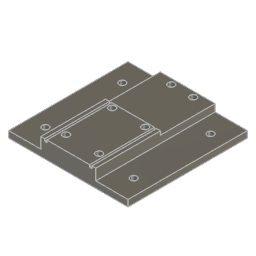
x_stage (Autodesk Fusion 360 design; units mm, degrees)
part number: 2026-04-23-15-36-49-562
Autodesk Fusion 360 part; units mm, degrees
note: some values were not read from the file. Chosen so that the rebuilt part matches the saved one: which face or edge a step refers to. Set by a fixed rule: which sketch regions a step uses.
sketch "Sketch1" plane through (0, 0, 0) normal (0, 0, 1) x (1, 0, 0)
  line L0 (-27.2, 27.2) -> (27.2, 27.2)
  line L1 (27.2, 27.2) -> (27.2, -27.2)
  line L2 (27.2, -27.2) -> (-27.2, -27.2)
  line L3 (-27.2, -27.2) -> (-27.2, 27.2)
  line L4 (-27.2, 27.2) -> (27.2, -27.2) construction
  line L5 (27.2, 27.2) -> (-27.2, -27.2) construction
  circle A0 centre (-20.1, 17.5) radius 1.5
  circle A1 centre (-20.1, -17.5) radius 1.5
  circle A2 centre (20.1, 17.5) radius 1.5
  circle A3 centre (20.1, -17.5) radius 1.5
  circle A4 centre (-4, 24.95) radius 1.5
  circle A5 centre (4, 24.95) radius 1.5
  circle A6 centre (-4, 7.95) radius 1.5
  circle A7 centre (4, 7.95) radius 1.5
  circle A8 centre (0, 10.7) radius 1.5
  dimension "d1" = 54.4
  dimension "d2" = 3
  dimension "d3" = 35
  dimension "d4" = 9.7
  dimension "d9" = 3
  dimension "d10" = 24.95
  dimension "d11" = 4
  dimension "d12" = 4
  dimension "d19" = 7.1
  dimension "d20" = 7.1
  dimension "d21" = 17
  dimension "d22" = 16.5
  dimension "d23" = 3
  constraint horizontal L0
  constraint perpendicular L0 L1
  constraint parallel L0 L2
  constraint parallel L1 L3
  constraint coincident L4 origin
  constraint coincident L5 origin
  constraint equal L0 L3
  constraint vertical A0.centre A1.centre
  constraint horizontal A1.centre A3.centre
  constraint vertical A2.centre A3.centre
  constraint horizontal A0.centre A2.centre
  constraint equal A0 A1
  constraint equal A1 A3
  constraint equal A2 A3
  constraint equal A4 A5
  constraint horizontal A4.centre A5.centre
  constraint vertical A5.centre A7.centre
  constraint vertical A4.centre A6.centre
  constraint equal A4 A6
  constraint equal A6 A7
  constraint horizontal A6.centre A7.centre
  constraint vertical origin A8.centre
  measures "d1" distance of L0.start L0.end
  measures "d2" diameter of A0
  measures "d3" distance of A0.centre A1.centre
  measures "d4" distance of L0 A0.centre
  measures "d9" diameter of A4
  measures "d10" vertical distance of origin A4.centre
  measures "d11" horizontal distance of origin A4.centre
  measures "d12" horizontal distance of origin A5.centre
  measures "d19" distance of L3 A0.centre
  measures "d20" distance of L1 A2.centre
  measures "d21" distance of A4.centre A6.centre
  measures "d22" distance of L0 A8.centre
  measures "d23" diameter of A8
extrude "Extrude1" add sketch "Sketch1" along normal blind 3 contours L0 L1 L2 L3 | A4 | A5 | A6 | A7 | A8
sketch "Sketch2" plane through (0, 0, 3) normal (0, 0, 1) x (-1, 0, 0)
  circle A0 centre (-20.1, 17.5) radius 1.5
  circle A1 centre (20.1, -17.5) radius 1.5
  circle A2 centre (20.1, 17.5) radius 1.5
  circle A3 centre (-20.1, -17.5) radius 1.5
  line L0 (27.2, 27.2) -> (-27.2, 27.2)
  line L1 (-27.2, 27.2) -> (-27.2, -27.2)
  line L2 (-27.2, -27.2) -> (27.2, -27.2)
  line L3 (27.2, -27.2) -> (27.2, 27.2)
  line L4 (12.5, -27.2) -> (-12.5, -27.2)
  line L5 (-12.5, -27.2) -> (-12.5, 27.2)
  line L6 (-12.5, 27.2) -> (12.5, 27.2)
  line L7 (12.5, 27.2) -> (12.5, -27.2)
  line L8 (12.5, -27.2) -> (-12.5, 27.2) construction
  line L9 (-12.5, -27.2) -> (12.5, 27.2) construction
  dimension "d13" = 25
  constraint horizontal L4
  constraint perpendicular L4 L5
  constraint parallel L4 L6
  constraint parallel L5 L7
  constraint coincident L8 origin
  constraint coincident L9 origin
  constraint coincident L2 L4.start
  measures "d13" distance of L4.start L4.end
extrude "Extrude2" add sketch "Sketch2" along normal blind 3 contours L0 L2 L4 L5 L6 L7
sketch "Sketch5" plane through (0, 0, 6) normal (0, 0, 1) x (-1, 0, 0)
  line L0 (12.5, 27.2) -> (-12.5, 27.2)
  line L1 (-12.5, 27.2) -> (-12.5, -27.2)
  line L2 (-12.5, -27.2) -> (12.5, -27.2)
  line L3 (12.5, -27.2) -> (12.5, 27.2)
  circle A0 centre (7.5, -0.3) radius 1.5
  circle A1 centre (-7.5, -0.3) radius 1.5
  circle A2 centre (7.5, 20.7) radius 1.5
  circle A3 centre (-7.5, 20.7) radius 1.5
  circle A4 centre (5, -24.7) radius 1.5
  circle A5 centre (-5, -24.7) radius 1.5
  circle A6 centre (5, -10.7) radius 1.5
  circle A7 centre (-5, -10.7) radius 1.5
  dimension "d27" = 15
  dimension "d28" = 21
  dimension "d29" = 3
  dimension "d31" = 7.5
  dimension "d34" = 10
  dimension "d35" = 14
  dimension "d36" = 3
  dimension "d37" = 5
  dimension "d38" = 2.5
  dimension "d49" = 26.9
  constraint vertical A0.centre A2.centre
  constraint horizontal A0.centre A1.centre
  constraint horizontal A2.centre A3.centre
  constraint vertical A1.centre A3.centre
  constraint equal A2 A3
  constraint equal A0 A2
  constraint equal A0 A1
  constraint vertical A4.centre A6.centre
  constraint horizontal A6.centre A7.centre
  constraint vertical A5.centre A7.centre
  constraint horizontal A4.centre A5.centre
  constraint equal A4 A5
  constraint equal A5 A7
  constraint equal A6 A7
  measures "d27" distance of A0.centre A1.centre
  measures "d28" distance of A0.centre A2.centre
  measures "d29" diameter of A0
  measures "d31" horizontal distance of origin A2.centre
  measures "d34" distance of A4.centre A5.centre
  measures "d35" vertical distance of A4.centre A6.centre
  measures "d36" diameter of A4
  measures "d37" horizontal distance of origin A4.centre
  measures "d38" distance of L2 A4.centre
  measures "d49" distance of L2 A0.centre
extrude "Extrude5" cut sketch "Sketch5" against normal blind 3 contours A0 | A1 | A2 | A3 | A4 | A5
sketch "Sketch6" plane through (0, 0, 6) normal (0, 0, 1) x (-1, 0, 0)
  line L0 (12.5, 27.2) -> (-12.5, 27.2)
  line L1 (-12.5, 27.2) -> (-12.5, -27.2)
  line L2 (-12.5, -27.2) -> (12.5, -27.2)
  line L3 (12.5, -27.2) -> (12.5, 27.2)
  circle A0 centre (5, -24.7) radius 1.5
  circle A1 centre (7.5, 20.7) radius 1.5
  circle A2 centre (7.5, -0.3) radius 1.5
  circle A3 centre (-5, -24.7) radius 1.5
  circle A4 centre (-7.5, 20.7) radius 1.5
  circle A5 centre (-7.5, -0.3) radius 1.5
  line L4 (12.5, 27.2) -> (-12.5, 27.2)
  line L5 (-12.5, 27.2) -> (-12.5, -2.3)
  line L6 (-12.5, -2.3) -> (12.5, -2.3)
  line L7 (12.5, -2.3) -> (12.5, 27.2)
  dimension "d39" = 29.5
  constraint horizontal L4
  constraint vertical L5
  constraint horizontal L6
  constraint vertical L7
  constraint coincident L1 L5.end
  constraint coincident L0.start L3.end
  measures "d39" distance of L0.start L6.end
extrude "Extrude6" add sketch "Sketch6" along normal blind 2 contours L0 L1 L3 L4 L5 L6 L7
extrude "Extrude8" add 1 faces at (1.484, 9.3012, 6) along direction (0, 0, 1) blind 0.3
sketch "Sketch8" plane through (0, 0, 8) normal (0, 0, 1) x (-1, 0, 0)
  circle A0 centre (7.5, -0.3) radius 1.5
  circle A1 centre (7.5, 20.7) radius 1.5
  circle A2 centre (-7.5, 20.7) radius 1.5
  circle A3 centre (-7.5, -0.3) radius 1.5
  line L0 (12.5, -2.3) -> (12.5, 27.2)
  line L1 (12.5, 27.2) -> (-12.5, 27.2)
  line L2 (-12.5, 27.2) -> (-12.5, -2.3)
  line L3 (-12.5, -2.3) -> (12.5, -2.3)
  line L4 (10.73, -2.3) -> (9.73, -2.3)
  line L5 (9.73, -2.3) -> (9.73, 27.2)
  line L6 (9.73, 27.2) -> (10.73, 27.2)
  line L7 (10.73, 27.2) -> (10.73, -2.3)
  line L8 (-9.73, -2.3) -> (-10.73, -2.3)
  line L9 (-10.73, -2.3) -> (-10.73, 27.2)
  line L10 (-10.73, 27.2) -> (-9.73, 27.2)
  line L11 (-9.73, 27.2) -> (-9.73, -2.3)
  dimension "d52" = 1
  dimension "d53" = 1.77
  dimension "d54" = 1.77
  constraint horizontal L4
  constraint vertical L5
  constraint horizontal L6
  constraint vertical L7
  constraint coincident L1 L5.end
  constraint coincident L3 L4.start
  constraint horizontal L8
  constraint vertical L9
  constraint horizontal L10
  constraint vertical L11
  constraint coincident L1 L9.end
  constraint coincident L3 L8.start
  constraint equal L4 L8
  measures "d52" distance of L4.start L4.end
  measures "d53" distance of L0 L7
  measures "d54" distance of L2 L9
extrude "Extrude9" cut sketch "Sketch8" against normal blind 1 contours L1 L3 L4 L5 L6 L7 | L1 L3 L8 L9 L10 L11
sketch "Sketch9" plane through (0, 0, 0) normal (0, 0, -1) x (1, 0, 0)
  circle A0 centre (20.1, 17.5) radius 1.5
  circle A1 centre (-20.1, 17.5) radius 1.5
  circle A2 centre (20.1, -17.5) radius 1.5
  circle A3 centre (-20.1, -17.5) radius 1.5
  line L0 (27.2, 27.2) -> (-27.2, 27.2)
  line L1 (-27.2, 27.2) -> (-27.2, -27.2)
  line L2 (-27.2, -27.2) -> (27.2, -27.2)
  line L3 (27.2, -27.2) -> (27.2, 27.2)
  line L4 (20.2, 15.2) -> (34.2, 15.2)
  arc A4 (34.2, 15.2) -> (34.2, 27.2) centre (34.2, 21.2) ccw
  line L5 (34.2, 27.2) -> (20.2, 27.2)
  arc A5 (20.2, 27.2) -> (20.2, 15.2) centre (20.2, 21.2) ccw
  line L6 (20.2, 21.2) -> (34.2, 21.2) construction
  circle A6 centre (34.2, 21.2) radius 3.125
  line L7 (0, 0) -> (0, -11.2612) construction
  line L8 (0, 0) -> (-11.04, 0) construction
  line L9 (0, 0) -> (0, -11.2612) construction
  circle A7 centre (-34.2, 21.2) radius 3.125
  arc A8 (-20.2, 15.2) -> (-20.2, 27.2) centre (-20.2, 21.2) ccw
  arc A9 (-34.2, 27.2) -> (-34.2, 15.2) centre (-34.2, 21.2) ccw
  line L10 (-34.2, 27.2) -> (-20.2, 27.2)
  line L11 (-20.2, 21.2) -> (-34.2, 21.2) construction
  line L12 (-20.2, 15.2) -> (-34.2, 15.2)
  circle A10 centre (-20.1, 17.5) radius 1.5
  line L13 (20.2, -21.2) -> (34.2, -21.2) construction
  line L14 (34.2, -27.2) -> (20.2, -27.2)
  arc A11 (34.2, -27.2) -> (34.2, -15.2) centre (34.2, -21.2) ccw
  arc A12 (20.2, -15.2) -> (20.2, -27.2) centre (20.2, -21.2) ccw
  line L15 (20.2, -15.2) -> (34.2, -15.2)
  circle A13 centre (20.1, -17.5) radius 1.5
  circle A14 centre (34.2, -21.2) radius 3.125
  line L16 (-20.2, -15.2) -> (-34.2, -15.2)
  arc A15 (-20.2, -27.2) -> (-20.2, -15.2) centre (-20.2, -21.2) ccw
  arc A16 (-34.2, -15.2) -> (-34.2, -27.2) centre (-34.2, -21.2) ccw
  circle A17 centre (-34.2, -21.2) radius 3.125
  circle A18 centre (-20.1, -17.5) radius 1.5
  line L17 (-20.2, -21.2) -> (-34.2, -21.2) construction
  line L18 (-34.2, -27.2) -> (-20.2, -27.2)
  circle A19 centre (-20.1, -17.5) radius 1.5
  point P0 (27.2, 21.2)
  point P1 (-27.2, 27.2)
  point P2 (-27.2, 21.2)
  point P3 (27.2, -27.2)
  point P4 (27.2, -21.2)
  point P5 (-27.2, -21.2)
  point P6 (-27.2, -27.2)
  point P7 (-27.2, -27.2)
  dimension "d62" = 6
  dimension "d63" = 6.25
  dimension "d64" = 6
  dimension "d65" = 7
  constraint tangent L4 A4
  constraint tangent A4 L5
  constraint parallel L4 L5
  constraint tangent L5 A5
  constraint tangent L4 A5
  constraint perpendicular L3 L6
  constraint coincident L3 P0
  constraint midpoint L6 P0
  constraint concentric A4 A6
  constraint coincident L7.start L8.start
  constraint vertical L7
  constraint perpendicular L7 L8
  constraint symmetric A0 L7 A10
  constraint symmetric L0.start L7 P1
  constraint symmetric L4.start L7 A8.start
  constraint symmetric L4.end L7 A9.end
  constraint symmetric A4.end L7 A9.start
  constraint symmetric L5.end L7 A8.end
  constraint symmetric A4 L7 A9
  constraint symmetric A5 L7 A8
  constraint symmetric P0 L7 P2
  constraint symmetric A6 L7 A7
  constraint symmetric L8.start L7 L9.start
  constraint symmetric L9.end L7 L7.end
  constraint symmetric A0 L8 A13
  constraint symmetric A1 L8 A19
  constraint symmetric L0.start L8 P3
  constraint symmetric P1 L8 P7
  constraint symmetric L4.start L8 A12.start
  constraint symmetric L4.end L8 A11.end
  constraint symmetric A4.end L8 L14.start
  constraint symmetric L5.end L8 L14.end
  constraint symmetric A4 L8 A11
  constraint symmetric A5 L8 A12
  constraint symmetric P0 L8 P4
  constraint symmetric A6 L8 A14
  constraint symmetric L8 A8.end A15.start
  constraint symmetric L8 A9.start A16.end
  constraint symmetric L8 P1 P7
  constraint symmetric L8 A8.start L16.start
  constraint symmetric L8 A9.end L16.end
  constraint symmetric L8 P2 P5
  constraint symmetric L8 A7 A17
  constraint symmetric L8 A8 A15
  constraint symmetric L8 A9 A16
  constraint symmetric L8 A10 A18
  measures "d62" radius of A4
  measures "d63" diameter of A6
  measures "d64" distance of L0 P0
  measures "d65" distance of L3 L4.end
extrude "Extrude10" [rolled back] along distance -3 taper angle 0
extrude "Extrude11" [rolled back] side1offset 0 taper angle 0
fillet "Fillet2" [rolled back] radius 2
ref_plane "WorkPlane1" through (0, 0, 1.5) normal (-1, 0, 0) x (0, -1, 0)
sketch "Sketch7" plane through (0, 0, 0) normal (-1, 0, 0) x (0, -1, 0)
  line L0 (27.2, 0) -> (27.2, 8.1)
  line L1 (27.2, 8.1) -> (17.2, 8.1)
  line L2 (17.2, 8.1) -> (9.1, 0)
  line L3 (9.1, 0) -> (27.2, 0)
  line L4 (-2.3, 8.1) -> (27.2, 8.1)
  line L5 (27.2, 3) -> (12.1, 3)
  line L6 (12.1, 3) -> (12.1, 0)
  point P0 (27.2, 8.1)
  point P1 (27.2, 0)
  dimension "d42" = 10
  dimension "d43" = 45
  dimension "d46" = 3
  constraint vertical L0
  constraint perpendicular L0 L1
  constraint horizontal L3
  constraint coincident P0 L0.end
  constraint coincident L0.start L3.end
  constraint coincident L0 L5.start
  constraint coincident L2 L5.end
  constraint perpendicular L0 L5
  constraint coincident L3 L6.end
  constraint perpendicular L3 L6
  measures "d42" distance of P0 L1.end
  measures "d43" angle of L2 L4
  measures "d46" distance of L3 L5
extrude "Extrude7" [suppressed]
sketch "Sketch4" plane through (0, 0, 0) normal (0, 0, -1) x (1, 0, 0)
  circle A0 centre (20.4, 17.5) radius 1.5
  circle A1 centre (0, -11) radius 1.5
  circle A2 centre (-5, -9.3) radius 1.5
  circle A3 centre (5, -9.3) radius 1.5
  circle A4 centre (-20.4, -17.5) radius 1.5
  circle A5 centre (20.4, -17.5) radius 1.5
  circle A6 centre (-5, -25) radius 1.5
  circle A7 centre (5, -25) radius 1.5
  line L0 (27.5, 27.5) -> (-27.5, 27.5)
  line L1 (-27.5, 27.5) -> (-27.5, -27.5)
  line L2 (-27.5, -27.5) -> (27.5, -27.5)
  line L3 (27.5, -27.5) -> (27.5, 27.5)
  circle A8 centre (-20.4, 17.5) radius 1.5
  circle A9 centre (0, -11) radius 2.5
  dimension "d24" = 5
  constraint concentric A1 A9
  measures "d24" diameter of A9
extrude "Extrude4" [suppressed]
sketch "Sketch3" plane through (0, 0, 6) normal (0, 0, 1) x (-1, 0, 0)
  circle A0 centre (-5, -20) radius 1.5
  circle A1 centre (5, -20) radius 1.5
  line L0 (10.3, 25) -> (-10.3, 25)
  line L1 (-10.3, 25) -> (-10.3, -25)
  line L2 (-10.3, -25) -> (10.3, -25)
  line L3 (10.3, -25) -> (10.3, 25)
  line L4 (10.3, 25) -> (-10.3, 25)
  line L5 (-10.3, 25) -> (-10.3, 20)
  line L6 (-10.3, 20) -> (10.3, 20)
  line L7 (10.3, 20) -> (10.3, 25)
  dimension "d16" = 5
  constraint horizontal L4
  constraint vertical L5
  constraint horizontal L6
  constraint vertical L7
  constraint coincident L1 L5.end
  constraint coincident L0.start L3.end
  measures "d16" distance of L0.end L5.end
extrude "Extrude3" [suppressed]
equation "d4 = ( d1 - d3 ) / 2"
equation "d5 = 26 mm + 1.9 mm - 2.5 mm"
equation "d10 = 25 mm - 0.95 mm + 1.2 mm - 0.3 mm"
equation "d12 = d11"
equation "d19 = d20"
equation "d22 = 14 mm + 2.5 mm"
equation "d23 = d9"
equation "d31 = d27 / 2"
equation "d37 = d34 / 2"
equation "d64 = d62"
